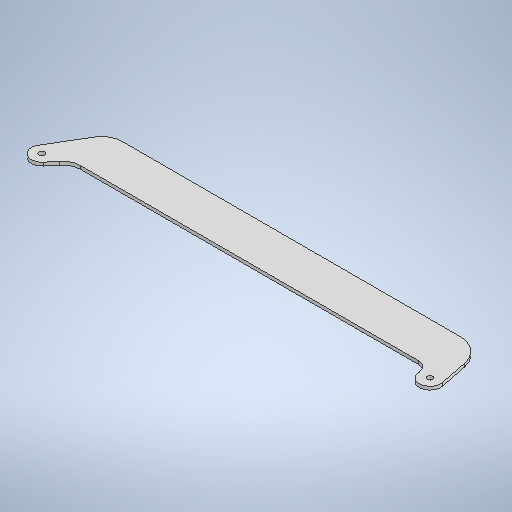
# Autodesk Inventor part: A3P1
Saved by Autodesk Inventor 2025.2 (Build 292293000, 293)
## iProperties
Created: 2025-05-22
Part Number: A3P1
Material: Generic
Document SubType Name: Sheet Metal
Designer: Admin
Density: 1 g/cm^3
Sheet Metal Rule: Default
Appearance: Default
Author: Admin
Autodesk Inventor part; units mm, degrees
ref_plane "YZ Plane" through (0, 0, 0) normal (1, 0, 0) x (0, 1, 0)
ref_plane "XZ Plane" through (0, 0, 0) normal (0, 1, 0) x (-1, 0, 0)
ref_plane "XY Plane" through (0, 0, 0) normal (0, 0, 1) x (1, 0, 0)
sketch "Sketch1" plane through (0, 0, 0) normal (0, 1, 0) x (-1, 0, 0)
  arc A0 (4.6831, -2.7877) -> (-4.2282, 3.4387) centre (0, 0) ccw
  line L0 (4.6831, -2.7877) -> (-6.0873, -20.8805)
  line L1 (-4.2282, 3.4387) -> (-7.9464, -1.1331)
  arc A1 (-15.3196, -26.129) -> (-6.0873, -20.8805) centre (-15.3196, -15.3847) ccw
  arc A2 (-15.3196, -4.6405) -> (-7.9464, -1.1331) centre (-15.3196, 4.8633) ccw
  line L2 (-15.3196, -26.129) -> (-189.4823, -26.129)
  line L3 (-15.3196, -4.6405) -> (-189.4823, -4.6405)
  arc A3 (-194.5547, 0.2259) -> (-205.3394, -1.0922) centre (-200, 0) ccw
  arc A4 (-194.5547, 0.2259) -> (-189.4823, -4.6405) centre (-189.4823, 0.4363) ccw
  arc A5 (-202.3696, -15.6109) -> (-189.4823, -26.129) centre (-189.4823, -12.9748) ccw
  line L4 (-202.3696, -15.6109) -> (-205.3394, -1.0922)
  point P0 (-6.0873, 1.1528)
  point P1 (-10.0096, -24.7251)
  point P2 (-0.7021, -11.8341)
  dimension "d0" = 10.9
  dimension "d1" = 10.9
  dimension "d2" = 200
  dimension "d3" = 0
  dimension "d6" = 0
  dimension "d7" = 0
  dimension "d8" = 0
  dimension "d9" = 174.1627
  dimension "d10" = 9.3075
  dimension "d11" = 13.1542
  constraints: 14 point on circle, 11 tangent, 10 end point, 6 centre point, 2 horizontal, 2 midpoint, 1 coincident
  measures "d0" diameter of A0
  measures "d1" diameter of A3
  measures "d2" distance of A3.centre point (0, 0)
  measures "d3" vertical distance of A3.centre point (0, 0)
  measures "d6" horizontal distance of L3.start L2.start
  measures "d7" horizontal distance of point (-6.087, 1.153) L0.end
  measures "d8" horizontal distance of L3.end L2.end
  measures "d9" distance of L2.start L2.end
  measures "d10" horizontal distance of point (-10.01, -24.725) point (-0.702, -11.834)
  measures "d11" radius of A5
extrude "Extrusion1" add sketch "Sketch1" along normal blind 1.7
sketch "Sketch2" plane through (0, 1.7, 0) normal (0, 1, 0) x (1, 0, 0)
  arc A0 (-4.6831, 2.7877) -> (4.2282, -3.4387) centre (0, 0) ccw projected
  circle A1 centre (0, 0) radius 1.5
  arc A2 (194.5547, -0.2259) -> (205.3394, 1.0922) centre (200, 0) ccw projected
  circle A3 centre (200, 0) radius 1.5
  dimension "d14" = 3
  dimension "d15" = 3
  constraints: 2 centre point, 2 coincident
  measures "d14" diameter of A3
  measures "d15" diameter of A1
extrude "Extrusion2" cut sketch "Sketch2" against normal blind 1.7
equation "\"BendRadius\" = Thickness"
equation "\"BendReliefWidth\" = Thickness"
equation "\"BendReliefDepth\" = 0.5 * Thickness"
equation "\"CornerReliefSize\" = 4 * Thickness"
equation "\"MinimumRemnant\" = 2 * Thickness"
equation "\"TransitionRadius\" = BendRadius"
equation "\"JacobiRadiusSize\" = BendRadius"
equation "\"GapSize\" = Thickness"
equation "\"Thickness\" = 3.048"
body "Solid1"
